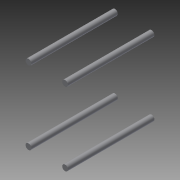
# Autodesk Inventor part: table
Saved by Autodesk Inventor 2015 (Build 190159000, 159)
## iProperties
Created: 2014-05-21
Part Number: table
Material: Generic
Document SubType Name: Modeling
Designer: jad211
Density: 1 g/cm^3
Appearance: Default
Author: jad211
Autodesk Inventor part; units mm, degrees
ref_plane "YZ Plane" through (0, 0, 0) normal (1, 0, 0) x (0, 1, 0)
ref_plane "XZ Plane" through (0, 0, 0) normal (0, 1, 0) x (-1, 0, 0)
ref_plane "XY Plane" through (0, 0, 0) normal (0, 0, 1) x (1, 0, 0)
sketch "Sketch1" plane through (0, 0, 0) normal (0, 1, 0) x (-1, 0, 0)
  circle A0 centre (0, 0) radius 3
  circle A1 centre (38.1, 0.0388) radius 3
  circle A2 centre (0, -76.2) radius 3
  circle A3 centre (38.1, -76.1612) radius 3
  line L0 (0, 0) -> (39.4176, 0) construction
  dimension "d0" = 6
  dimension "d3" = 6
  dimension "d4" = 6
  dimension "d5" = 6
  dimension "d6" = 38.1
  dimension "d7" = 76.2
  dimension "d8" = 38.1
  dimension "d9" = 76.2
  constraints: 4 centre point, 2 end point, 1 coincident, 1 horizontal
  measures "d0" diameter of A0
  measures "d3" diameter of A1
  measures "d4" diameter of A3
  measures "d5" diameter of A2
  measures "d6" distance of A1.centre point (0, 0)
  measures "d7" distance of A2.centre point (0, 0)
  measures "d8" distance of A3.centre A2.centre
  measures "d9" distance of A1.centre A3.centre
extrude "Extrusion2" add sketch "Sketch1" along normal blind 90
equation "\"d3\" = d0"
equation "\"d4\" = d3"
equation "\"d5\" = d4"
equation "\"d7\" = 2 * d6"
equation "\"d8\" = d6"
equation "\"d9\" = d7"
body "Solid2"
